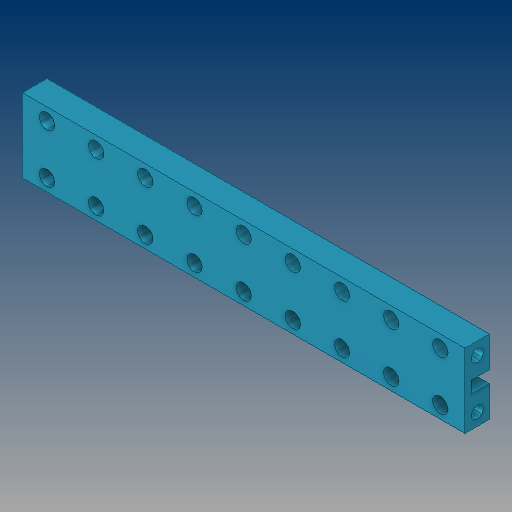
# Autodesk Inventor part: Beam0824-144-Blue
Saved by Autodesk Inventor 2017 (Build 210142000, 142)
## iProperties
Created: 2017-03-13
Part Number: Beam0824-144-Blue
Material: Aluminum 6061
Document SubType Name: Modeling
Designer: zallen
Density: 2.7 g/cm^3
Appearance: Aluminum - Flat
Catalog Web Link: http://www.makeblock.com/beam0824-144-blue-4-pack
Mass: 57.1415 g
Surface Area: 130.362 cm^2
Volume: 21.1635 cm^3
Author: zallen
Autodesk Inventor part; units mm, degrees
ref_plane "YZ Plane" through (0, 0, 0) normal (1, 0, 0) x (0, 1, 0)
ref_plane "XZ Plane" through (0, 0, 0) normal (0, 1, 0) x (-1, 0, 0)
ref_plane "XY Plane" through (0, 0, 0) normal (0, 0, 1) x (1, 0, 0)
sketch "Sketch1" plane through (0, 0, 0) normal (0, 0, 1) x (1, 0, 0)
  line L0 (144, 0) -> (0, 0)
  line L1 (0, 0) -> (0, 24)
  line L2 (0, 24) -> (144, 24)
  line L3 (144, 24) -> (144, 0)
  point P0 (0, 0)
  dimension "d0" = 144
  dimension "d1" = 24
  constraints: 8 end point, 2 parallel, 1 coincident, 1 horizontal, 1 perpendicular
  measures "d0" distance of L1.end L2.end
  measures "d1" distance of L0.end L1.end
extrude "Extrusion1" add sketch "Sketch1" along normal blind 8
sketch "Sketch5" plane through (0, 0, 8) normal (0, 0, 1) x (1, 0, 0)
  circle A0 centre (136, 20) radius 2.5
  line L0 (144, 20) -> (0, 20) construction
  line L1 (136, 24) -> (136, 0) construction
  line L2 (144, 24) -> (0, 24) construction
  line L3 (0, 0) -> (144, 0) construction
  line L4 (0, 24) -> (144, 24) construction
  line L5 (144, 24) -> (144, 0) construction
  line L6 (144, 0) -> (0, 0) construction
  line L7 (0, 0) -> (0, 24) construction
  circle A1 centre (120, 20) radius 2.5
  circle A2 centre (104, 20) radius 2.5
  circle A3 centre (88, 20) radius 2.5
  circle A4 centre (72, 20) radius 2.5
  circle A5 centre (56, 20) radius 2.5
  circle A6 centre (40, 20) radius 2.5
  circle A7 centre (24, 20) radius 2.5
  circle A8 centre (8, 20) radius 2.5
  circle A9 centre (136, 4) radius 2.5
  circle A10 centre (120, 4) radius 2.5
  circle A11 centre (104, 4) radius 2.5
  circle A12 centre (88, 4) radius 2.5
  circle A13 centre (72, 4) radius 2.5
  circle A14 centre (56, 4) radius 2.5
  circle A15 centre (40, 4) radius 2.5
  circle A16 centre (24, 4) radius 2.5
  circle A17 centre (8, 4) radius 2.5
  dimension "d30" = 5
  dimension "d83" = 4
  dimension "d84" = 8
  dimension "d87" = 16
  dimension "d90" = 16
  constraints: 18 centre point, 12 end point, 2 horizontal, 2 parallel, 2 vertical, 1 perpendicular, 1 point on line, 34 other
  measures "d30" diameter of A0
  measures "d83" distance between parallel lines of L0 L2
  measures "d84" distance between parallel lines of L5 L1
  measures "d87" distance of A0.centre A1.centre
  measures "d90" distance of A0.centre A9.centre
extrude "Extrusion8" cut sketch "Sketch5" against normal through all
sketch "Sketch9" plane through (144, 0, 0) normal (1, 0, 0) x (0, 0, -1)
  circle A0 centre (-4, 20) radius 2
  circle A1 centre (-4, 4) radius 2
  line L0 (0, 0) -> (-8, 0) projected
  line L1 (0, 24) -> (-8, 24) construction
  line L2 (-8, 24) -> (0, 24) construction
  line L3 (0, 24) -> (0, 0) construction
  line L4 (0, 0) -> (-8, 0) construction
  line L5 (-8, 0) -> (-8, 24) construction
  point P0 (0, 0)
  dimension "d95" = 4
  dimension "d96" = 4
  dimension "d97" = 4
  dimension "d98" = 4
  dimension "d99" = 4
  dimension "d100" = 4
  constraints: 8 end point, 2 centre point, 2 parallel, 1 horizontal, 1 perpendicular
  measures "d95" diameter of A0
  measures "d96" diameter of A1
  measures "d97" distance from line of A1.centre L0
  measures "d98" distance from line of L3 A0.centre
  measures "d99" distance from line of L3 A1.centre
  measures "d100" distance from line of L1 A0.centre
extrude "Extrusion9" cut sketch "Sketch9" against normal blind 4
sketch "Sketch10" plane through (0, 0, 0) normal (-1, 0, 0) x (0, 0, 1)
  line L0 (0, 24) -> (0, 0) construction
  line L1 (0, 24) -> (8, 24) construction
  line L2 (8, 24) -> (8, 0) construction
  line L3 (8, 0) -> (0, 0) construction
  line L4 (0, 0) -> (0, 24) construction
  circle A0 centre (4, 20) radius 2
  circle A1 centre (4, 4) radius 2
  point P0 (0, 0)
  dimension "d107" = 4
  dimension "d108" = 4
  dimension "d109" = 4
  dimension "d110" = 4
  dimension "d111" = 4
  dimension "d112" = 4
  constraints: 8 end point, 2 centre point, 2 parallel, 1 horizontal, 1 perpendicular
  measures "d107" diameter of A0
  measures "d108" diameter of A1
  measures "d109" distance from line of L1 A0.centre
  measures "d110" distance from line of L2 A0.centre
  measures "d111" distance from line of L3 A1.centre
  measures "d112" distance from line of L2 A1.centre
extrude "Extrusion10" cut sketch "Sketch10" against normal blind 4
sketch "Sketch11" plane through (0, 0, 0) normal (0, 0, -1) x (-1, 0, 0)
  line L0 (-144, 24) -> (-144, 0) projected
  line L1 (-144, 14) -> (0, 14)
  line L2 (0, 14) -> (0, 10)
  line L3 (0, 10) -> (-144, 10)
  line L4 (-144, 10) -> (-144, 14)
  line L5 (0, 24) -> (-144, 24) projected
  line L6 (-144, 0) -> (0, 0) projected
  point P0 (0, 0)
  dimension "d119" = 10
  dimension "d120" = 10
  dimension "d121" = 144
  constraints: 8 end point, 2 parallel, 1 horizontal, 1 perpendicular, 1 point on line
  measures "d119" distance between parallel lines of L5 L1
  measures "d120" distance between parallel lines of L6 L3
  measures "d121" distance between parallel lines of L0 L2
extrude "Extrusion11" cut sketch "Sketch11" against normal blind 6
body "Solid1"
